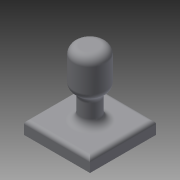
# Autodesk Inventor part: SMI Stamp Holder
Saved by Autodesk Inventor 2015 (Build 190159000, 159)
## iProperties
Created: 2014-08-17
Part Number: SMI Stamp Holder
Material: Generic
Document SubType Name: Modeling
Designer: Chris
Density: 1 g/cm^3
Appearance: Default
Author: Chris
Autodesk Inventor part; units mm, degrees
ref_plane "YZ Plane" through (0, 0, 0) normal (1, 0, 0) x (0, 1, 0)
ref_plane "XZ Plane" through (0, 0, 0) normal (0, 1, 0) x (-1, 0, 0)
ref_plane "XY Plane" through (0, 0, 0) normal (0, 0, 1) x (1, 0, 0)
sketch "Sketch2" plane through (0, 0, 0) normal (0, 1, 0) x (-1, 0, 0)
  line L0 (18.3186, 20.469) -> (-22.6814, 20.469)
  line L1 (-22.6814, 20.469) -> (-22.6814, -20.531)
  line L2 (-22.6814, -20.531) -> (18.3186, -20.531)
  line L3 (18.3186, -20.531) -> (18.3186, 20.469)
  line L4 (-27.6814, 25.469) -> (23.3186, 25.469)
  line L5 (23.3186, 25.469) -> (23.3186, -25.531)
  line L6 (23.3186, -25.531) -> (-27.6814, -25.531)
  line L7 (-27.6814, -25.531) -> (-27.6814, 25.469)
  line L8 (-22.6814, 20.469) -> (18.3186, 20.469)
  line L9 (18.3186, 20.469) -> (18.3186, -20.531)
  line L10 (18.3186, -20.531) -> (-22.6814, -20.531)
  line L11 (-22.6814, -20.531) -> (-22.6814, 20.469)
  line L12 (-22.6814, 20.469) -> (18.3186, 20.469)
  line L13 (18.3186, 20.469) -> (18.3186, -20.531)
  line L14 (18.3186, -20.531) -> (-22.6814, -20.531)
  line L15 (-22.6814, -20.531) -> (-22.6814, 20.469)
  point P0 (0, 0)
  dimension "d0" = 41
  dimension "d1" = 41
  dimension "d6" = 5
  constraints: 32 end point, 8 parallel, 4 perpendicular, 3 horizontal, 3 other
  measures "d0" distance of L2.end L0.start
  measures "d1" distance of L1.end L2.end
  measures "d6" distance between parallel lines of L0 L4
extrude "Extrusion1" add sketch "Sketch2" along normal blind 10 contours L3 L2 L1 L0 | L4 L5 L6 L7
sketch "Sketch5" plane through (0, 0, 0) normal (0, -1, 0) x (1, 0, 0)
  line L0 (27.6814, 25.469) -> (-23.3186, 25.469)
  line L1 (-23.3186, 25.469) -> (-23.3186, -25.531)
  line L2 (-23.3186, -25.531) -> (27.6814, -25.531)
  line L3 (27.6814, -25.531) -> (27.6814, 25.469)
  line L4 (-18.3186, 20.469) -> (22.6814, 20.469)
  line L5 (22.6814, 20.469) -> (22.6814, -20.531)
  line L6 (22.6814, -20.531) -> (-18.3186, -20.531)
  line L7 (-18.3186, -20.531) -> (-18.3186, 20.469)
  point P0 (0, 0)
  dimension "d10" = 5
  constraints: 16 end point, 4 parallel, 2 perpendicular, 1 horizontal, 3 other
  measures "d10" distance between parallel lines of L0 L4
extrude "Extrusion2" cut sketch "Sketch5" against normal blind 4 contours L4 L5 L6 L7
fillet "Fillet1" radius 3 4 edges at (-23.3186, 10, -0.031) (2.1814, 10, 25.469) (27.6814, 10, -0.031) (2.1814, 10, -25.531)
sketch "Sketch6" plane through (0, 10, 0) normal (0, 1, 0) x (1, 0, 0)
  circle A0 centre (2.1814, 0.031) radius 7.5
  line L0 (-23.3186, 25.531) -> (27.6814, 25.531) projected
  line L1 (27.6814, -25.469) -> (-23.3186, -25.469) projected
  point P0 (0, 0)
  dimension "d14" = 15
  constraints: 1 centre point
  measures "d14" diameter of A0
extrude "Extrusion3" add sketch "Sketch6" along normal blind 50
sketch "Sketch7" plane through (2.1814, 60, -0.031) normal (0, 1, 0) x (1, 0, 0)
  circle A0 centre (0, 0) radius 12.5
  point P0 (-2.1814, -0.031)
  dimension "d17" = 25
  constraints: 1 centre point
  measures "d17" diameter of A0
extrude "Extrusion4" add sketch "Sketch7" against normal blind 30
fillet "Fillet2" radius 6 1 edges at (-10.3186, 60, -0.031)
fillet "Fillet3" radius 6 1 edges at (-10.3186, 30, -0.031)
fillet "Fillet4" radius 6 1 edges at (-5.3186, 30, -0.031)
fillet "Fillet5" radius 6 1 edges at (-5.3186, 10, -0.031)
body "Solid1"
